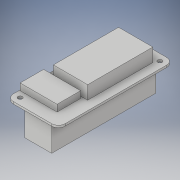
# Autodesk Inventor part: PCB
Saved by Autodesk Inventor 2019 (Build 230136000, 136)
## iProperties
Created: 2019-04-30
Part Number: PCB
Material: Generic
Document SubType Name: Modeling
Designer: Henry
Density: 1 g/cm^3
Appearance: Default
Author: Henry
Autodesk Inventor part; units mm, degrees
ref_plane "YZ Plane" through (0, 0, 0) normal (1, 0, 0) x (0, 1, 0)
ref_plane "XZ Plane" through (0, 0, 0) normal (0, 1, 0) x (-1, 0, 0)
ref_plane "XY Plane" through (0, 0, 0) normal (0, 0, 1) x (1, 0, 0)
sketch "Sketch1" plane through (0, 0, 0) normal (0, 1, 0) x (-1, 0, 0)
  line L0 (5, 0) -> (33.5, 0)
  line L1 (38.5, -5) -> (38.5, -80.5)
  line L2 (33.5, -85.5) -> (5, -85.5)
  line L3 (0, -80.5) -> (0, -5)
  arc A0 (38.5, -5) -> (33.5, 0) centre (33.5, -5) ccw
  arc A1 (33.5, -85.5) -> (38.5, -80.5) centre (33.5, -80.5) ccw
  arc A2 (0, -80.5) -> (5, -85.5) centre (5, -80.5) ccw
  arc A3 (5, 0) -> (0, -5) centre (5, -5) ccw
  point P0 (0, 0)
  point P1 (38.5, -85.5)
  point P2 (38.5, 0)
  point P3 (0, -85.5)
  dimension "d0" = 38.5
  dimension "d1" = 85.5
  dimension "d2" = 5
  dimension "d3" = 5
  dimension "d4" = 5
  dimension "d5" = 5
  constraints: 8 end point, 8 point on circle, 8 point on line, 8 tangent, 4 centre point, 2 parallel, 1 horizontal, 1 perpendicular
  measures "d0" distance of point (38.5, -85.5) point (0, -85.5)
  measures "d1" distance of point (38.5, 0) point (38.5, -85.5)
  measures "d2" radius of A0
  measures "d3" radius of A1
  measures "d4" radius of A2
  measures "d5" radius of A3
extrude "Extrusion1" add sketch "Sketch1" along normal blind 1.6
sketch "Sketch2" plane through (0, 1.6, 0) normal (0, 1, 0) x (1, 0, 0)
  arc A0 (-5, 0) -> (0, 5) centre (-5, 5) ccw projected
  arc A1 (0, 80.5) -> (-5, 85.5) centre (-5, 80.5) ccw projected
  circle A2 centre (-5, 80.5) radius 1.6
  arc A3 (-33.5, 85.5) -> (-38.5, 80.5) centre (-33.5, 80.5) ccw projected
  circle A4 centre (-33.5, 80.5) radius 1.6
  arc A5 (-38.5, 5) -> (-33.5, 0) centre (-33.5, 5) ccw projected
  circle A6 centre (-33.5, 5) radius 1.6
  point P0 (0, 0)
  dimension "d9" = 3.2
  dimension "d10" = 3.2
  dimension "d11" = 3.2
  constraints: 3 centre point, 3 coincident
  measures "d9" diameter of A2
  measures "d10" diameter of A4
  measures "d11" diameter of A6
extrude "Extrusion2" cut sketch "Sketch2" against normal blind 35
sketch "Sketch4" plane through (0, 0, 0) normal (0, -1, 0) x (1, 0, 0)
  line L0 (0, 0) -> (-9.5, 0)
  line L1 (-9.5, 0) -> (-9.5, -4.5)
  line L2 (-9.5, -4.5) -> (0, -4.5)
  line L3 (0, -4.5) -> (0, 0)
  line L4 (-9.5, -4.5) -> (-29.5, -4.5)
  line L5 (-29.5, -4.5) -> (-29.5, -82)
  line L6 (-29.5, -82) -> (-9.5, -82)
  line L7 (-9.5, -82) -> (-9.5, -4.5)
  dimension "d14" = 9.5
  dimension "d15" = 4.5
  dimension "d16" = 20
  dimension "d17" = 77.5
  constraints: 16 end point, 4 parallel, 2 horizontal, 2 perpendicular
  measures "d14" distance of L2.end L1.end
  measures "d15" distance of L1.end L0.end
  measures "d16" distance of L6.end L5.end
  measures "d17" distance of L5.end L4.end
extrude "Extrusion3" add sketch "Sketch4" along normal blind 22 contours L7 L6 L5 L4
sketch "Sketch5" plane through (0, 1.6, 0) normal (0, 1, 0) x (1, 0, 0)
  line L0 (0, 0) -> (-10.5, 0)
  line L1 (-10.5, 0) -> (-10.5, 9.5)
  line L2 (-10.5, 9.5) -> (0, 9.5)
  line L3 (0, 9.5) -> (0, 0)
  line L4 (-10.5, 9.5) -> (-38, 9.5)
  line L5 (-38, 9.5) -> (-38, 27)
  line L6 (-38, 27) -> (-10.5, 27)
  line L7 (-10.5, 27) -> (-10.5, 9.5)
  dimension "d20" = 10.5
  dimension "d21" = 9.5
  dimension "d22" = 27.5
  dimension "d23" = 17.5
  constraints: 16 end point, 4 parallel, 2 horizontal, 2 perpendicular
  measures "d20" distance of L1.end L2.end
  measures "d21" distance of L0.end L1.end
  measures "d22" distance of L5.end L6.end
  measures "d23" distance of L4.end L5.end
extrude "Extrusion4" add sketch "Sketch5" along normal blind 5 contours L4 L5 L6 L7
sketch "Sketch6" plane through (0, 1.6, 0) normal (0, 1, 0) x (1, 0, 0)
  line L0 (0, 0) -> (-6.75, 0)
  line L1 (-6.75, 0) -> (-6.75, 28.5)
  line L2 (-6.75, 28.5) -> (0, 28.5)
  line L3 (0, 28.5) -> (0, 0)
  line L4 (-6.75, 28.5) -> (-32.25, 28.5)
  line L5 (-32.25, 28.5) -> (-32.25, 77)
  line L6 (-32.25, 77) -> (-6.75, 77)
  line L7 (-6.75, 77) -> (-6.75, 28.5)
  dimension "d26" = 6.75
  dimension "d27" = 28.5
  dimension "d28" = 25.5
  dimension "d29" = 48.5
  constraints: 16 end point, 4 parallel, 2 horizontal, 2 perpendicular
  measures "d26" distance of L1.end L2.end
  measures "d27" distance of L0.end L1.end
  measures "d28" distance of L5.end L6.end
  measures "d29" distance of L4.end L5.end
extrude "Extrusion5" add sketch "Sketch6" along normal blind 10 contours L4 L5 L6 L7
body "Solid1"
